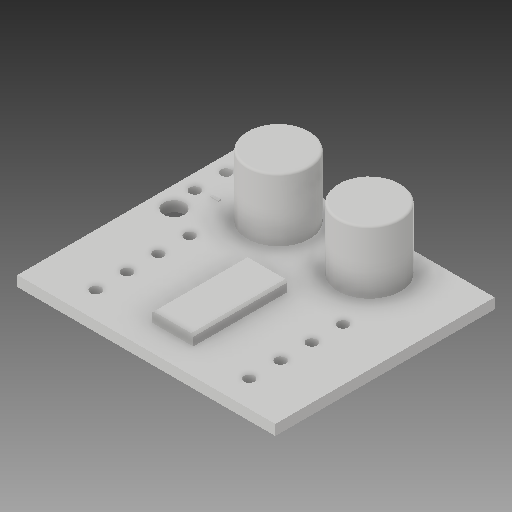
# Autodesk Inventor part: L298N_CPY
Saved by Autodesk Inventor 2019 (Build 230136000, 136)
## iProperties
Created: 2018-12-15
Part Number: L298N_CPY
Material: Generic
Document SubType Name: Modeling
Designer: Filip
Density: 1 g/cm^3
Appearance: Default
Author: Filip
Autodesk Inventor part; units mm, degrees
ref_plane "YZ Plane" through (0, 0, 0) normal (1, 0, 0) x (0, 1, 0)
ref_plane "XZ Plane" through (0, 0, 0) normal (0, 1, 0) x (-1, 0, 0)
ref_plane "XY Plane" through (0, 0, 0) normal (0, 0, 1) x (1, 0, 0)
sketch "Sketch1" plane through (0, 0, 0) normal (0, 1, 0) x (-1, 0, 0)
  line L0 (-12.35, 10.5) -> (12.35, 10.5)
  line L1 (12.35, 10.5) -> (12.35, -10.5)
  line L2 (12.35, -10.5) -> (-12.35, -10.5)
  line L3 (-12.35, -10.5) -> (-12.35, 10.5)
  line L4 (-12.35, 10.5) -> (12.35, -10.5) construction
  line L5 (12.35, 10.5) -> (-12.35, -10.5) construction
  point P0 (0, 0)
  dimension "d0" = 21
  dimension "d1" = 24.7
  constraints: 12 end point, 2 midpoint, 2 parallel, 1 horizontal, 1 perpendicular
  measures "d0" distance of L0.end L1.end
  measures "d1" distance of L0.start L0.end
extrude "Extrusion1" add sketch "Sketch1" along normal blind 1
sketch "Sketch2" plane through (0, 1, 0) normal (0, 1, 0) x (1, 0, 0)
  circle A0 centre (-10.35, 2.5) radius 1
  line L0 (12.35, 10.5) -> (-12.35, 10.5) projected
  line L1 (-12.35, 10.5) -> (-12.35, -10.5) projected
  point P0 (0, 0)
  dimension "d4" = 2
  dimension "d5" = 8
  dimension "d6" = 2
  constraints: 1 centre point
  measures "d4" diameter of A0
  measures "d5" distance from line of L0 A0.centre
  measures "d6" distance from line of L1 A0.centre
extrude "Extrusion2" cut sketch "Sketch2" against normal blind 1
sketch "Sketch3" plane through (0, 1, 0) normal (0, 1, 0) x (1, 0, 0)
  circle A0 centre (-4.35, 6.5) radius 3
  line L0 (-12.35, 10.5) -> (-12.35, -10.5) projected
  line L1 (12.35, 10.5) -> (-12.35, 10.5) projected
  line L2 (0, 0) -> (0, 10.5) construction
  circle A1 centre (4.35, 6.5) radius 3
  dimension "d9" = 6
  dimension "d10" = 8
  dimension "d11" = 4
  constraints: 2 centre point, 2 end point, 1 midpoint, 1 symmetric about line, 1 other
  measures "d9" diameter of A0
  measures "d10" distance from line of L0 A0.centre
  measures "d11" distance from line of L1 A0.centre
extrude "Extrusion3" add sketch "Sketch3" along normal blind 6
fillet "Fillet1" radius 0.2 2 edges at (-7.35, 7, -6.5) (1.35, 7, -6.5)
sketch "Sketch4" plane through (0, 1, 0) normal (0, 1, 0) x (1, 0, 0)
  circle A0 centre (-7.35, 1) radius 0.5
  circle A1 centre (-7.35, -2) radius 0.5
  circle A2 centre (-10.35, 2.5) radius 1 projected
  line L0 (-10.35, 1.5) -> (-7.35, 1.5) construction
  circle A3 centre (-7.35, -5) radius 0.5
  circle A4 centre (-7.35, -8) radius 0.5
  circle A5 centre (-4.35, 6.5) radius 3 projected
  line L1 (-7.35, 6.5) -> (-7.35, 1.5) construction
  line L2 (0, 0) -> (0, -10.5851) construction
  circle A6 centre (7.35, 1) radius 0.5
  circle A7 centre (7.35, -2) radius 0.5
  circle A8 centre (7.35, -5) radius 0.5
  circle A9 centre (7.35, -8) radius 0.5
  dimension "d15" = 1
  dimension "d16" = 1
  dimension "d17" = 1
  dimension "d18" = 1
  dimension "d19" = 3
  dimension "d20" = 3
  dimension "d21" = 3
  constraints: 7 centre point, 6 end point, 5 vertical alignment, 4 symmetric about line, 3 horizontal, 3 vertical, 1 horizontal alignment, 8 other
  measures "d16" diameter of A1
  measures "d17" diameter of A3
  measures "d18" diameter of A4
  measures "d19" distance of A1.centre point (-7.35, 1)
  measures "d20" distance of A3.centre A1.centre
  measures "d21" distance of A4.centre A3.centre
extrude "Extrusion4" cut sketch "Sketch4" against normal blind 1 contours A0 | A1 | A3 | A4 | A6 | A7 | A8 | A9
sketch "Sketch5" plane through (0, 1, 0) normal (0, 1, 0) x (1, 0, 0)
  line L0 (-2, 1) -> (2, 1)
  line L1 (2, 1) -> (2, -8)
  line L2 (2, -8) -> (-2, -8)
  line L3 (-2, -8) -> (-2, 1)
  circle A0 centre (-7.35, 1) radius 0.5 projected
  point P0 (0, 0)
  point P1 (0, 1)
  dimension "d26" = 4
  dimension "d27" = 9
  constraints: 8 end point, 2 parallel, 1 horizontal, 1 horizontal alignment, 1 midpoint, 1 perpendicular, 1 vertical alignment
  measures "d26" distance of L0.start L0.end
  measures "d27" distance of L2.end L0.start
extrude "Extrusion5" add sketch "Sketch5" along normal blind 1 contours L0 L1 L2 L3
chamfer "Chamfer1" distance 0.2 angle 45 2 edges at (2, 2, 3.5) (-2, 2, 3.5)
sketch "Sketch6" plane through (0, 1, 0) normal (0, 1, 0) x (1, 0, 0)
  circle A0 centre (-10.85, 8) radius 0.5
  circle A1 centre (-10.85, 5) radius 0.5
  line L0 (12.35, 10.5) -> (-12.35, 10.5) projected
  line L1 (-12.35, 10.5) -> (-12.35, -10.5) projected
  point P0 (0, 0)
  dimension "d33" = 1
  dimension "d34" = 1
  dimension "d35" = 2.5
  dimension "d36" = 1.5
  dimension "d37" = 3
  constraints: 2 centre point, 1 vertical alignment
  measures "d33" diameter of A0
  measures "d34" diameter of A1
  measures "d35" distance from line of L0 A0.centre
  measures "d36" distance from line of L1 A0.centre
  measures "d37" distance of A1.centre A0.centre
extrude "Extrusion6" cut sketch "Sketch6" against normal blind 1
sketch "Sketch7" plane through (0, 1, 0) normal (0, 1, 0) x (1, 0, 0)
  line L0 (-9.7434, 8.3067) -> (-6.693, 8.3067) construction
  line L1 (-6.693, 8.3067) -> (-6.693, 5.9132) construction
  line L2 (-6.693, 5.9132) -> (-9.7434, 5.9132) construction
  line L3 (-9.7434, 5.9132) -> (-9.7434, 8.3067) construction
  line L4 (-9.6683, 5.4228) -> (-8.67, 5.4228) construction
  line L5 (-8.67, 5.4228) -> (-8.67, 5.1797) construction
  line L6 (-8.67, 5.1797) -> (-9.6683, 5.1797) construction
  line L7 (-9.6683, 5.1797) -> (-9.6683, 5.4228) construction
  line L8 (-8.848, 7.8602) -> (-9.1867, 7.8602)
  line L9 (-9.1867, 7.8602) -> (-9.1867, 7.5214)
  line L10 (-9.1867, 7.5214) -> (-9.2985, 7.5214)
  line L11 (-9.2985, 7.5214) -> (-9.2985, 7.8602)
  line L12 (-9.2985, 7.8602) -> (-9.6373, 7.8602)
  line L13 (-9.6373, 7.8602) -> (-9.6373, 7.9679)
  line L14 (-9.6373, 7.9679) -> (-9.2985, 7.9679)
  line L15 (-9.2985, 7.9679) -> (-9.2985, 8.3067)
  line L16 (-9.2985, 8.3067) -> (-9.1867, 8.3067)
  line L17 (-9.1867, 8.3067) -> (-9.1867, 7.9679)
  line L18 (-9.1867, 7.9679) -> (-8.848, 7.9679)
  line L19 (-8.848, 7.9679) -> (-8.848, 7.8602)
  line L20 (-8.7899, 5.1797) -> (-9.5468, 5.1797)
  line L21 (-9.5468, 5.1797) -> (-9.5468, 5.4228)
  line L22 (-9.5468, 5.4228) -> (-8.7899, 5.4228)
  line L23 (-8.7899, 5.4228) -> (-8.7899, 5.1797)
  point P0 (0, 0)
  constraints: 4 other
emboss "Emboss1" sketch "Sketch7" operation add depth 0.1 direction (0, -1, 0)
body "Solid1"
